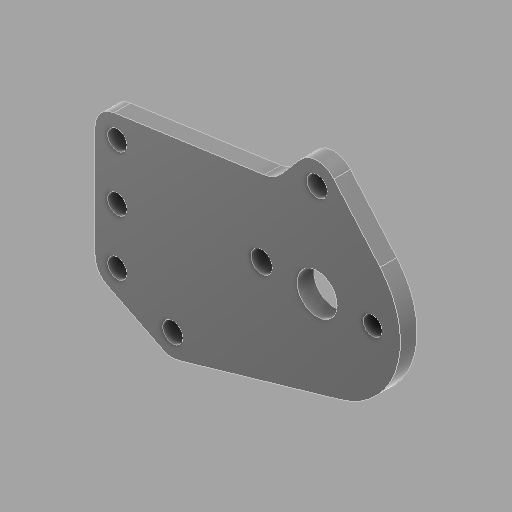
# Autodesk Inventor part: Stage2
Saved by Autodesk Inventor 2026.1 (Build 301233000, 233)
## iProperties
Created: 2025-10-04
Part Number: Stage2
Material: Plastic, Opaque Black
Document SubType Name: Modeling
Designer: Teddy
Density: 0.952 g/cm^3
Appearance: Smooth - Black
Author: Teddy
Autodesk Inventor part; units mm, degrees
ref_plane "YZ Plane" through (0, 0, 0) normal (1, 0, 0) x (0, 1, 0)
ref_plane "XZ Plane" through (0, 0, 0) normal (0, 1, 0) x (-1, 0, 0)
ref_plane "XY Plane" through (0, 0, 0) normal (0, 0, 1) x (1, 0, 0)
ref_plane "Work Plane1" through (0, 0, 0) normal (0, 0, 1) x (1, 0, 0)
sketch "Sketch1" plane through (0, 0, 0) normal (0, 0, 1) x (1, 0, 0)
  circle A0 centre (1.1498, -25.4) radius 2.1844 projected
  circle A1 centre (1.1498, -38.1) radius 2.1844 projected
  circle A2 centre (1.1498, -50.8) radius 2.1844 projected
  arc A3 (42.6103, -14.4523) -> (32.4711, -20.5468) centre (46.8698, -33.02) ccw construction
  line L0 (1.1498, -25.4) -> (1.1498, -50.8) construction
  line L1 (-3.9302, -25.4) -> (-3.9302, -50.8)
  line L2 (6.2298, -50.8) -> (6.2298, -25.4)
  arc A4 (6.2298, -25.4) -> (-3.9302, -25.4) centre (1.1498, -25.4) ccw
  arc A5 (-3.9302, -50.8) -> (6.2298, -50.8) centre (1.1498, -50.8) ccw
  line L3 (1.5665, -55.8629) -> (48.4323, -52.0058) construction
  line L4 (44.1924, -14.1591) -> (42.5701, -14.3894) construction
  circle A6 centre (46.8698, -33.02) radius 4.572
  circle A7 centre (59.5698, -33.02) radius 2.1209 projected
  circle A8 centre (34.1698, -33.02) radius 2.4209 projected
  circle A9 centre (13.8498, -57.1457) radius 2.286
  arc A10 (11.5792, -61.69) -> (15.2652, -62.0245) centre (13.8498, -57.1457) ccw
  line L5 (-1.1208, -55.3443) -> (11.5792, -61.69)
  line L6 (15.2652, -62.0245) -> (52.1776, -51.3156)
  circle A11 centre (46.8698, -11.684) radius 2.286
  arc A12 (42.5701, -14.3894) -> (50.7094, -8.3578) centre (46.8698, -11.684) ccw construction
  line L7 (50.7094, -8.3578) -> (61.2684, -20.5468)
  line L8 (43.0301, -8.3578) -> (38.6923, -13.3652)
  line L9 (37.137, -15.1606) -> (32.4711, -20.5468) construction
  line L10 (42.5701, -14.3894) -> (37.137, -15.1606) construction
  arc A13 (44.1924, -14.1591) -> (42.6103, -14.4523) centre (46.8698, -33.02) ccw construction
  arc A14 (51.1292, -14.4523) -> (44.1924, -14.1591) centre (46.8698, -33.02) ccw construction
  arc A15 (43.0301, -8.3578) -> (42.5701, -14.3894) centre (46.8698, -11.684) ccw construction
  arc A16 (50.7094, -8.3578) -> (43.0301, -8.3578) centre (46.8698, -11.684) ccw
  line L11 (34.7852, -15.4945) -> (0.4358, -20.3704)
  arc A17 (32.4711, -20.5468) -> (48.4323, -52.0058) centre (46.8698, -33.02) ccw construction
  arc A18 (48.4323, -52.0058) -> (52.1776, -51.3156) centre (46.8698, -33.02) ccw construction
  arc A19 (52.1776, -51.3156) -> (61.2684, -20.5468) centre (46.8698, -33.02) ccw
  arc A20 (9.141, -55.2395) -> (11.5792, -61.69) centre (13.8498, -57.1457) ccw construction
  arc A21 (15.2652, -62.0245) -> (9.141, -55.2395) centre (13.8498, -57.1457) ccw construction
  arc A22 (34.7852, -15.4945) -> (38.6923, -13.3652) centre (33.8928, -9.2075) ccw
  arc A23 (61.2684, -20.5468) -> (51.1292, -14.4523) centre (46.8698, -33.02) ccw construction
  point P0 (0, 0)
  point P1 (1.1498, -38.1)
  dimension "d0" = 38.1
  dimension "d1" = 10.16
  dimension "d2" = 45.72
  dimension "d6" = 9.144
  dimension "d8" = 7.62
  dimension "d9" = 4.572
  dimension "d10" = 10.16
  dimension "d11" = 12.7
  dimension "d12" = 4.572
  dimension "d13" = 10.16
  dimension "d14" = 6.35
  constraints: 54 tangent, 49 point on circle, 26 end point, 19 centre point, 4 point on line, 3 coincident, 1 midpoint, 1 parallel, 1 vertical, 1 vertical alignment
  measures "d0" diameter of A3
  measures "d1" diameter of A5
  measures "d2" horizontal distance of L0.start A3.centre
  measures "d6" diameter of A6
  measures "d8" vertical distance of L0.start A3.centre
  measures "d9" diameter of A9
  measures "d10" diameter of A10
  measures "d11" horizontal distance of L0.end A10.centre
  measures "d12" diameter of A11
  measures "d13" diameter of A12
  measures "d14" radius of A22
extrude "Extrusion1" add sketch "Sketch1" along normal blind 3.81
body "Solid1"
